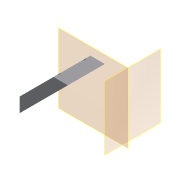
# Autodesk Inventor part: 20_Cube_Insert_Kinematic_Mirrormount_45_base_part2
Saved by Autodesk Inventor 2019 (Build 230136000, 136)
## iProperties
Created: 2019-07-01
Part Number: 20_Cube_Insert_Kinematic_Mirrormount_45_base_part2
Material: Generic
Document SubType Name: Modeling
Designer: diederichbenedict
Density: 1 g/cm^3
Appearance: Default
Author: diederichbenedict
Autodesk Inventor part; units mm, degrees
ref_plane "YZ Plane" through (0, 0, 0) normal (1, 0, 0) x (0, 1, 0)
ref_plane "XZ Plane" through (0, 0, 0) normal (0, 1, 0) x (-1, 0, 0)
ref_plane "Work Plane1" through (0, 0, 10) normal (0, 0, 1) x (1, 0, 0)
sketch "Sketch1" plane through (0, 0, 10) normal (0, 0, 1) x (1, 0, 0)
  line L0 (-4.0299, -0.3538) -> (-2.2322, 1.4439) construction
  arc A0 (-1.4439, 2.2322) -> (-2.2322, 1.4439) centre (-0.9299, 0.9299) ccw construction
  line L1 (-1.4439, 2.2322) -> (0.3538, 4.0299) construction
  line L2 (-37.8299, 42.8299) -> (-37.8299, 37.8299) construction
  line L3 (-37.8299, 37.8299) -> (-42.9208, 37.8299) construction
  line L4 (-37.8299, 42.2137) -> (-37.8299, 45.8299) construction
  line L5 (-37.8299, 45.8299) -> (-4.0299, 45.8299) construction
  line L6 (-4.0299, 45.8299) -> (-4.0299, 42.2137) construction
  line L7 (-4.0299, 4.0299) -> (0.3538, 4.0299) projected
  circle A1 centre (-20.9299, 20.9299) radius 17.5 projected
  line L8 (-20.9299, 58.9723) -> (17.1124, 20.9299) construction
  line L9 (17.1124, 20.9299) -> (-20.9299, -17.1124) construction
  line L10 (-20.9299, -17.1124) -> (-58.9723, 20.9299) construction
  line L11 (-58.9723, 20.9299) -> (-20.9299, 58.9723) construction
  line L12 (-20.9299, 58.9723) -> (-20.9299, -17.1124) construction
  line L13 (17.1124, 20.9299) -> (-58.9723, 20.9299) construction
  line L14 (-20.9299, 58.9723) -> (32.8701, 58.9723) construction
  line L15 (-43.4299, 43.4299) -> (1.5701, 43.4299) construction
  line L16 (1.5701, 43.4299) -> (1.5701, -1.5701) construction
  line L17 (1.5701, -1.5701) -> (-43.4299, -1.5701) construction
  line L18 (-43.4299, -1.5701) -> (-43.4299, 43.4299) construction
  line L19 (-43.4299, 43.4299) -> (1.5701, -1.5701) construction
  line L20 (1.5701, 43.4299) -> (-43.4299, -1.5701) construction
  line L21 (-43.4299, 5.3876) -> (-43.4299, 36.4723)
  line L22 (-43.4299, 36.4723) -> (-36.4723, 43.4299)
  line L23 (-36.4723, 43.4299) -> (-5.3876, 43.4299)
  line L24 (-5.3876, 43.4299) -> (1.5701, 36.4723)
  line L25 (1.5701, 36.4723) -> (1.5701, 5.3876)
  line L26 (1.5701, 5.3876) -> (-5.3876, -1.5701)
  line L27 (-5.3876, -1.5701) -> (-36.4723, -1.5701)
  line L28 (-36.4723, -1.5701) -> (-43.4299, 5.3876)
  line L29 (-4.0299, 42.2137) -> (-37.8299, 42.2137) projected
  line L30 (-4.0299, -0.3538) -> (-4.0299, 4.0299) projected
  circle A2 centre (-20.9299, 20.9299) radius 1.4
  line L31 (-10.9299, 10.9299) -> (-30.9299, 10.9299) construction
  line L32 (-30.9299, 10.9299) -> (-30.9299, 30.9299) construction
  line L33 (-30.9299, 30.9299) -> (-10.9299, 30.9299) construction
  line L34 (-10.9299, 30.9299) -> (-10.9299, 10.9299) construction
  line L35 (-10.9299, 10.9299) -> (-30.9299, 30.9299) construction
  line L36 (-30.9299, 10.9299) -> (-10.9299, 30.9299) construction
  circle A3 centre (-30.9299, 30.9299) radius 1.4
  circle A4 centre (-30.9299, 10.9299) radius 1.4
  circle A5 centre (-10.9299, 10.9299) radius 1.4
  line L37 (-45.8299, 37.8299) -> (-42.0723, 37.8299) construction
  line L38 (-42.1723, 37.7299) -> (-45.8299, 37.7299)
  line L39 (-45.8299, 37.7299) -> (-45.8299, 4.1299)
  line L40 (-45.8299, 4.1299) -> (-42.1723, 4.1299)
  line L41 (-42.1723, 4.1299) -> (-42.1723, 37.7299)
  line L42 (-45.8299, 4.0299) -> (-42.0723, 4.0299) construction
  line L43 (-45.8299, 37.8299) -> (-42.0723, 37.8299) projected
  line L44 (-37.7299, 45.8299) -> (-4.1299, 45.8299)
  line L45 (-4.1299, 45.8299) -> (-4.1299, 42.1723)
  line L46 (-4.1299, 42.1723) -> (-37.7299, 42.1723)
  line L47 (-37.7299, 42.1723) -> (-37.7299, 45.8299)
  line L48 (0.4701, 37.8299) -> (0.4701, 4.0299) construction
  line L49 (0.4701, 4.0299) -> (3.9701, 4.0299) construction
  line L50 (3.9701, 37.8299) -> (3.9701, 4.0299) construction
  line L51 (0.4701, 37.8299) -> (3.9701, 37.8299) construction
  line L52 (-45.8299, -3.9701) -> (-4.0299, -3.9701) construction
  line L53 (0.3124, 37.7299) -> (3.9701, 37.7299)
  line L54 (3.9701, 37.7299) -> (3.9701, 4.1299)
  line L55 (3.9701, 4.1299) -> (0.3124, 4.1299)
  line L56 (0.3124, 4.1299) -> (0.3124, 37.7299)
  line L57 (-4.1713, -0.3538) -> (-37.7299, -0.3538)
  line L58 (-37.7299, -0.3538) -> (-37.7299, -3.9701)
  line L59 (-37.7299, -3.9701) -> (-4.1713, -3.9701)
  line L60 (-4.1713, -3.9701) -> (-4.1713, -0.3538)
  point P0 (-37.8299, 4.0299)
  dimension "d18" = 53.8
  dimension "d19" = 45
  dimension "d20" = 53.8
  dimension "d21" = 45
  dimension "d22" = 45
  dimension "d30" = 20
  dimension "d31" = 20
  dimension "d32" = 2.8
  dimension "d33" = 2.8
  dimension "d34" = 2.8
  dimension "d35" = 2.8
  dimension "d36" = 0.1
  dimension "d37" = 0.1
  dimension "d38" = 0.1
  dimension "d39" = 0.1
  constraints: 86 end point, 21 point on line, 14 parallel, 8 perpendicular, 7 horizontal, 7 midpoint, 4 centre point, 4 coincident, 1 equal length
  measures "d18" distance of L8.start L8.end
  measures "d19" angle of L8 L14
  measures "d20" distance of L8.end L9.end
  measures "d21" distance of L16.end L17.end
  measures "d22" distance of L15.end L16.end
  measures "d30" distance of L32.end L33.end
  measures "d31" distance of L31.end L32.end
  measures "d32" diameter of A3
  measures "d33" diameter of A4
  measures "d34" diameter of A5
  measures "d35" diameter of A2
  measures "d36" distance between parallel lines of L38 L43
  measures "d37" distance between parallel lines of L40 L42
  measures "d38" distance between parallel lines of L45 L6
  measures "d39" distance between parallel lines of L4 L47
extrude "Extrusion1" add sketch "Sketch1" along normal blind 5 contours L30 L26 L57 L28 L41 L22 L46 L24 L56 L7 | L7 L26 L30 | L56 L24 L25 L26 | L26 L25 L24 L53 L54 L55 | L60 L59 L58 L57 L28 L27 L26 | L26 L27 L28 L57 | L46 L22 L29 L24 | L24 L29 L45 | L40 L39 L38 L22 L21 L28 | L28 L21 L22 L41 | L29 L22 L23 L24 | L24 L23 L22 L29 L47 L44 L45 | L47 L29 L22 | A1 | A2 | A3 | A4 | A5
sketch "Sketch4" plane through (0, 0, 15) normal (0, 0, 1) x (1, 0, 0)
  line L0 (-37.7299, 42.1723) -> (-42.1723, 37.7299) projected
  line L1 (-42.1723, 37.7299) -> (-45.8299, 37.7299) projected
  line L2 (-45.8299, 37.7299) -> (-45.8299, 4.1299) projected
  line L3 (-45.8299, 4.1299) -> (-42.1723, 4.1299) projected
  line L4 (-42.1723, 4.1299) -> (-37.6885, -0.3538) projected
  line L5 (-37.6885, -0.3538) -> (-37.7299, -0.3538) projected
  line L6 (-37.7299, -0.3538) -> (-37.7299, -3.9701) projected
  line L7 (-37.7299, -3.9701) -> (-4.1713, -3.9701) projected
  line L8 (-4.1713, -3.9701) -> (-4.1713, -0.3538) projected
  line L9 (-4.1713, -0.3538) -> (0.3124, 4.1299) projected
  line L10 (0.3124, 4.1299) -> (3.9701, 4.1299) projected
  line L11 (3.9701, 4.1299) -> (3.9701, 37.7299) projected
  line L12 (3.9701, 37.7299) -> (0.3124, 37.7299) projected
  line L13 (0.3124, 37.7299) -> (-4.1299, 42.1723) projected
  line L14 (-4.1299, 42.1723) -> (-4.1299, 45.8299) projected
  line L15 (-4.1299, 45.8299) -> (-37.7299, 45.8299) projected
  line L16 (-37.7299, 45.8299) -> (-37.7299, 42.1723) projected
  line L17 (-45.8299, 37.7299) -> (-45.8299, 4.1299) projected
  line L18 (-45.8299, 7.911) -> (-7.911, 45.8299)
  line L19 (-45.8299, 7.911) -> (7.7955, 7.911) construction
  line L20 (-7.911, 45.8299) -> (-19.2247, 45.8299)
  line L21 (-4.1299, 45.8299) -> (-37.7299, 45.8299) projected
  line L22 (-19.2247, 45.8299) -> (-45.8299, 19.2247)
  line L23 (-45.8299, 7.911) -> (-45.8299, 19.2247)
  circle A0 centre (-40.9299, 0.9299) radius 1.1933 projected
  circle A1 centre (-0.9299, 40.9299) radius 1.4 projected
  line L24 (-40.9299, 0.9299) -> (-0.9299, 40.9299)
  line L25 (0.3124, 37.7299) -> (-4.1299, 42.1723) projected
  point P0 (0, 0)
  dimension "d40" = 45
  dimension "d41" = 8
  constraints: 12 end point, 4 point on line, 1 collinear, 1 equal length, 1 horizontal, 1 perpendicular
  measures "d40" angle of L19 L18
  measures "d41" distance between parallel lines of L22 L18
extrude "Extrusion4" add sketch "Sketch4" along normal blind 28 contours L15 L18 L2 L22
sketch "Sketch5" plane through (-45.8299, 19.2247, 15) normal (-0.7071068, 0.7071068, 0) x (-0.7071068, -0.7071068, 0)
  line L0 (0, 0) -> (-37.6254, 0) projected
  line L1 (0, 0) -> (0, 28) projected
  line L2 (-37.6254, 28) -> (0, 28) projected
  line L3 (-37.6254, 0) -> (-37.6254, 28) projected
  circle A0 centre (-18.8127, 9.1873) radius 18.8127
  line L4 (-6.8127, 24) -> (-36.8127, 24) construction
  line L5 (-36.8127, 24) -> (-36.8127, 4) construction
  line L6 (-36.8127, 4) -> (-6.8127, 4) construction
  line L7 (-6.8127, 4) -> (-6.8127, 24) construction
  line L8 (-6.8127, 24) -> (-36.8127, 4) construction
  line L9 (-36.8127, 24) -> (-6.8127, 4) construction
  point P0 (-18.8127, -15)
  point P1 (-21.8127, 14)
  dimension "d44" = 30
  dimension "d45" = 20
  constraints: 12 end point, 3 tangent, 2 midpoint, 2 parallel, 1 centre point, 1 horizontal, 1 perpendicular
  measures "d44" distance of L6.end L5.end
  measures "d45" distance of L5.end L4.end
hole "Hole1" at (-19.7994, 45.2552, 39) at (-19.7994, 45.2552, 19) at (-41.0126, 24.042, 39) at (-30.406, 34.6486, 29) direction (0.7071068, -0.7071068, 0) diameter 2.9 depth 12
sketch "Sketch6" plane through (-37.7299, -3.9701, 10) normal (0, -1, 0) x (1, 0, 0)
  circle A0 centre (-3.2, 36.9) radius 1.45 projected
  circle A1 centre (36.8, 36.9) radius 1.45 projected
  line L0 (-6.1, 0) -> (-6.1, 39.8) projected
  line L1 (-0.1, 0) -> (-6.1, 0) projected
  line L2 (-0.1, 33.8) -> (-0.1, 0) projected
  line L3 (33.7, 33.8) -> (-0.1, 33.8) projected
  line L4 (33.7, 33.8) -> (33.7, 0) projected
  line L5 (39.7, 0) -> (33.7, 0) projected
  line L6 (39.7, 39.8) -> (39.7, 0) projected
  line L7 (-6.1, 39.8) -> (39.7, 39.8) projected
  circle A2 centre (16.8, 16.9) radius 16.9
  circle A3 centre (16.8, 16.9) radius 14.9
  line L8 (-0.1, 16.9) -> (-0.1, 0)
  line L9 (0, 0) -> (33.5586, 0) projected
  line L10 (0.0414, 0) -> (-4.4423, 0) projected
  line L11 (33.5586, 0) -> (0.0414, 0)
  line L12 (33.7, 16.9) -> (33.5586, 0)
  point P0 (37.7299, -10)
  dimension "d53" = 2
  constraints: 6 end point, 4 tangent, 2 centre point, 2 midpoint, 2 point on circle, 1 perpendicular, 1 vertical
  measures "d53" radial gap between concentric circles of A2 A3
extrude "Extrusion5" cut sketch "Sketch6" against normal up to surface contours A3 surface through (-45.8299, 7.911, 15) normal (0.7071068, -0.7071068, 0)
ref_plane "Work Plane3" through (3.9701, 45.8299, 26) normal (1, 0, 0) x (0, -1, 0)
sketch "Sketch7" plane through (3.9701, 45.8299, 26) normal (1, 0, 0) x (0, -1, 0)
  line L0 (41.8, -17.8) -> (41.8, 16) projected
  line L1 (8, -17.8) -> (41.8, -17.8) projected
  line L2 (8, -17.8) -> (8, 16) projected
  circle A0 centre (24.9, -0.9) radius 16.9
  circle A1 centre (24.9, -0.9) radius 14.9
  point P0 (45.8299, 26)
  dimension "d56" = 2
  constraints: 3 tangent, 2 centre point
  measures "d56" radial gap between concentric circles of A0 A1
ref_plane "Work Plane4" through (-34.8055, 8.3289, 16.6138) normal (0.7071068, -0.7071068, 0) x (0.7071068, 0.7071068, 0)
extrude "Extrusion6" cut sketch "Sketch7" against normal up to surface contours A1 surface through (-45.8299, 7.911, 15) normal (0.7071068, -0.7071068, 0)
sketch "Sketch8" plane through (-45.8299, 19.2247, 15) normal (-0.7071068, 0.7071068, 0) x (-0.7071068, -0.7071068, 0)
  arc A0 (-37.6254, 2.7992) -> (-37.6254, 5.2008) centre (-36.8127, 4) ccw projected
  circle A1 centre (-36.8127, 4) radius 7.5
  point P0 (-18.8127, -15)
  dimension "d59" = 15
  constraints: 1 centre point, 1 coincident
  measures "d59" diameter of A1
extrude "Extrusion7" cut sketch "Sketch8" along normal blind 10
sketch "Sketch9" plane through (0, 0, 10) normal (0, 0, -1) x (-1, 0, 0)
  line L0 (45.8299, 19.2247) -> (24.2855, 40.7692) projected
  line L1 (41.7776, 11.9633) -> (26.8705, 26.8705) projected
  line L2 (26.8705, 26.8705) -> (11.9633, 41.7776) projected
  line L3 (19.2247, 45.8299) -> (24.2855, 40.7692) projected
  line L4 (7.911, 45.8299) -> (11.9633, 41.7776) projected
  line L5 (41.7776, 11.9633) -> (45.8299, 7.911) projected
  line L6 (15.1679, 38.5731) -> (20.8247, 44.2299) projected
  line L7 (13.1172, 40.6237) -> (18.3235, 45.8299) projected
  line L8 (34.3304, 19.4105) -> (39.9873, 25.0673) projected
  line L9 (36.3811, 17.3599) -> (42.0379, 23.0167) projected
  circle A0 centre (20.5065, 38.8913) radius 1.4
  line L10 (25.7745, 27.9665) -> (31.4313, 33.6233) projected
  line L11 (31.4313, 33.6233) -> (25.7745, 27.9665)
  line L12 (26.8705, 26.8705) -> (32.5273, 32.5273)
  circle A1 centre (38.8913, 20.5065) radius 1.4
  point P0 (0, 0)
  point P1 (34.7528, 24.7491)
  dimension "d62" = 2.8
  constraints: 5 point on line, 4 end point, 2 centre point, 1 perpendicular, 1 symmetric about line, 1 other
  measures "d62" diameter of A0
hole "Hole2" at (-20.5065, 38.8913, 10) at (-38.8913, 20.5065, 10) direction (0, 0, 1) diameter 2.8 depth 12 counterbore diameter 5.5 counterbore depth 3
sketch "Sketch11" plane through (0, 0, 43) normal (0, 0, 1) x (1, 0, 0)
  line L0 (-7.911, 45.8299) -> (-19.2247, 45.8299) projected
  line L1 (-19.2247, 45.8299) -> (-45.8299, 19.2247) projected
  line L2 (-45.8299, 19.2247) -> (-45.8299, 7.911) projected
  line L3 (-45.8299, 7.911) -> (-7.911, 45.8299) projected
  line L4 (-45.8299, 37.7299) -> (-45.8299, 19.2247) projected
  line L5 (-42.1723, 37.7299) -> (-45.8299, 37.7299) projected
  line L6 (-37.7299, 42.1723) -> (-42.1723, 37.7299) projected
  line L7 (-37.7299, 45.8299) -> (-37.7299, 42.1723) projected
  line L8 (-29.3463, 45.8299) -> (-37.7299, 45.8299) projected
  line L9 (-29.3463, 45.8299) -> (-19.2247, 45.8299) projected
  line L10 (-4.1299, 45.8299) -> (-7.911, 45.8299) projected
  line L11 (-4.1299, 42.1723) -> (-4.1299, 45.8299) projected
  line L12 (0.3124, 37.7299) -> (-4.1299, 42.1723) projected
  line L13 (3.9701, 37.7299) -> (0.3124, 37.7299) projected
  line L14 (3.9701, 29.8965) -> (3.9701, 11.9633) projected
  line L15 (3.9701, 29.8965) -> (3.9701, 37.7299) projected
  line L16 (-11.9633, -3.9701) -> (-4.1713, -3.9701) projected
  line L17 (-4.1713, -3.9701) -> (-4.1713, -0.3538) projected
  line L18 (-4.1713, -0.3538) -> (0.3124, 4.1299) projected
  line L19 (0.3124, 4.1299) -> (3.9701, 4.1299) projected
  line L20 (3.9701, 4.1299) -> (3.9701, 11.9633) projected
  line L21 (-11.9633, -3.9701) -> (-29.8965, -3.9701) projected
  line L22 (-37.7299, -3.9701) -> (-29.8965, -3.9701) projected
  line L23 (-37.7299, -0.3538) -> (-37.7299, -3.9701) projected
  line L24 (-45.8299, 7.911) -> (-7.911, 45.8299) projected
  line L25 (-45.8299, 7.911) -> (-7.911, 45.8299)
  line L26 (-45.8299, 7.911) -> (-45.8299, 4.1299) projected
  line L27 (-45.8299, 4.1299) -> (-42.1723, 4.1299) projected
  line L28 (-37.6885, -0.3538) -> (-37.7299, -0.3538) projected
  line L29 (-42.1723, 4.1299) -> (-37.6885, -0.3538) projected
  point P0 (0, 0)
  constraints: 2 end point, 1 collinear
extrude "Extrusion8" cut sketch "Sketch11" against normal through all contours L10 L11 L12 L13 L15 L14 L20 L19 L18 L17 L16 L21 L22 L23 L28 L29 L27 L26 L3 | L1 L4 L5 L6 L7 L8 L9
sketch "Sketch12" plane through (-45.8299, 19.2247, 10) normal (-0.7071068, 0.7071068, 0) x (-0.7071068, -0.7071068, 0)
  line L0 (-45.6254, 33) -> (-45.6254, 0) projected
  line L1 (8, 0) -> (8, 33) projected
  line L2 (-45.6254, 0) -> (8, 0)
  line L3 (8, 0) -> (8, 4)
  line L4 (8, 4) -> (-45.6254, 4)
  line L5 (-45.6254, 4) -> (-45.6254, 0)
  point P0 (-18.8127, -10)
  point P1 (45.6254, -4)
  point P2 (45.6254, -5)
  point P3 (-8, -5)
  point P4 (-8, -4)
  dimension "d73" = 4
  constraints: 8 end point, 2 parallel, 1 horizontal, 1 perpendicular, 3 other
  measures "d73" distance between parallel lines of L2 L4
extrude "Extrusion9" cut sketch "Sketch12" against normal blind 29
body "Solid1"
